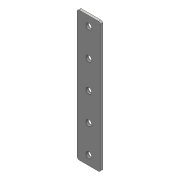
# Autodesk Inventor part: Connector
Saved by Autodesk Inventor 2016 (Build 200138000, 138)
## iProperties
Created: 2015-06-14
Part Number: Connector
Material: Generic
Document SubType Name: Sheet Metal
Designer: krosie
Density: 1 g/cm^3
Sheet Metal Rule: Default_mm
Appearance: Default
Author: krosie
Autodesk Inventor part; units mm, degrees
ref_plane "YZ Plane" through (0, 0, 0) normal (1, 0, 0) x (0, 1, 0)
ref_plane "XZ Plane" through (0, 0, 0) normal (0, 1, 0) x (-1, 0, 0)
ref_plane "XY Plane" through (0, 0, 0) normal (0, 0, 1) x (1, 0, 0)
sketch "Sketch1" plane through (0, 0, 0) normal (0, 1, 0) x (-1, 0, 0)
  line L0 (0, 0) -> (25, 0)
  line L1 (25, 0) -> (25, -140)
  line L2 (25, -140) -> (0, -140)
  line L3 (0, -140) -> (0, 0)
  circle A0 centre (12.5, -10) radius 3.05
  circle A1 centre (12.5, -70) radius 3.05
  circle A2 centre (12.5, -130) radius 3.05
  line L4 (25, -70) -> (0, -70) construction
  line L5 (12.5, 0) -> (12.5, -140) construction
  circle A3 centre (12.5, -40) radius 3.05
  circle A4 centre (12.5, -100) radius 3.05
  dimension "d0" = 25
  dimension "d1" = 140
  dimension "d2" = 6.1
  dimension "d3" = 6.1
  dimension "d4" = 6.1
  dimension "d5" = 10
  dimension "d6" = 10
  dimension "d7" = 6.1
  dimension "d8" = 6.1
  dimension "d9" = 30
  dimension "d10" = 30
  constraints: 12 end point, 7 midpoint, 5 centre point, 4 point on line, 2 parallel, 1 coincident, 1 horizontal, 1 perpendicular
  measures "d0" distance of L1.end L2.end
  measures "d1" distance of L0.end L1.end
  measures "d2" diameter of A0
  measures "d3" diameter of A1
  measures "d4" diameter of A2
  measures "d5" distance from line of L0 A0.centre
  measures "d6" distance from line of L2 A2.centre
  measures "d7" diameter of A3
  measures "d8" diameter of A4
  measures "d9" distance of A3.centre A0.centre
  measures "d10" distance of A2.centre A4.centre
extrude "Extrusion1" add sketch "Sketch1" along normal blind 2.5
fillet "Fillet1" radius 2 4 edges at (0, 1.25, 0) (-25, 1.25, 0) (0, 1.25, -140) (-25, 1.25, -140)
equation "\"BendRadius\" = Thickness"
equation "\"BendReliefWidth\" = Thickness"
equation "\"BendReliefDepth\" = 0.5 * Thickness"
equation "\"CornerReliefSize\" = 4 * Thickness"
equation "\"MinimumRemnant\" = 2 * Thickness"
equation "\"TransitionRadius\" = BendRadius"
equation "\"JacobiRadiusSize\" = BendRadius"
equation "\"GapSize\" = Thickness"
equation "\"Thickness\" = 0.5"
body "Solid1"
